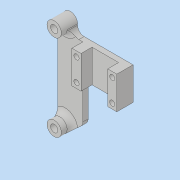
# Autodesk Inventor part: ribbonCableMount1
Saved by Autodesk Inventor 2017 (Build 210142000, 142)
## iProperties
Created: 2019-07-12
Part Number: ribbonCableMount1
Material: Generic
Document SubType Name: Modeling
Designer: techn
Density: 1 g/cm^3
Appearance: Default
Author: techn
Autodesk Inventor part; units mm, degrees
ref_plane "YZ Plane" through (0, 0, 0) normal (1, 0, 0) x (0, 1, 0)
ref_plane "XZ Plane" through (0, 0, 0) normal (0, 1, 0) x (-1, 0, 0)
ref_plane "XY Plane" through (0, 0, 0) normal (0, 0, 1) x (1, 0, 0)
sketch "Sketch1" plane through (0, 0, 0) normal (0, 0, 1) x (1, 0, 0)
  circle A0 centre (0, 0) radius 3.4925
  circle A1 centre (0, 41.91) radius 3.4925
  line L0 (0, 0) -> (-43.0857, 0) construction
  circle A2 centre (0, 41.91) radius 1.778
  circle A3 centre (0, 0) radius 1.778
  line L1 (3.4925, 41.91) -> (3.4925, 38.1)
  line L2 (3.4925, 38.1) -> (30.48, 38.1)
  line L3 (30.48, 38.1) -> (30.48, 22.225)
  line L4 (30.48, 22.225) -> (2.3101, -2.6193)
  line L5 (-3.4925, 41.91) -> (-3.4925, 0)
  dimension "d0" = 6.985
  dimension "d1" = 6.985
  dimension "d2" = 41.91
  dimension "d3" = 90
  dimension "d5" = 3.556
  dimension "d6" = 3.556
  dimension "d7" = 3.81
  dimension "d8" = 30.48
  dimension "d29" = 15.875
  constraints: 12 end point, 4 centre point, 4 point on circle, 4 tangent, 3 coincident, 2 perpendicular, 1 horizontal, 1 vertical
  measures "d0" diameter of A0
  measures "d1" diameter of A1
  measures "d2" distance of point (0, 0) A1.centre
  measures "d5" diameter of A2
  measures "d6" diameter of A3
  measures "d7" distance from line of L2 A1.centre
  measures "d8" distance from line of L3 A1.centre
  measures "d29" distance of L2.end L3.end
extrude "Extrusion1" add sketch "Sketch1" along normal blind 2.54
sketch "Sketch3" plane through (0, 0, 2.54) normal (0, 0, 1) x (1, 0, 0)
  circle A0 centre (0, 41.91) radius 1.778 construction
  circle A1 centre (0, 0) radius 1.778 construction
  arc A2 (-3.4925, 0) -> (2.3101, -2.6193) centre (0, 0) ccw construction
  line L0 (2.3101, -2.6193) -> (30.48, 22.225) construction
  line L1 (30.48, 22.225) -> (30.48, 38.1) construction
  line L2 (30.48, 38.1) -> (3.4925, 38.1) construction
  line L3 (3.4925, 38.1) -> (3.4925, 41.91) construction
  arc A3 (3.4925, 41.91) -> (-3.4925, 41.91) centre (0, 41.91) ccw construction
  line L4 (-3.4925, 41.91) -> (-3.4925, 0) construction
  line L5 (30.48, 22.225) -> (30.48, 38.1) projected
  line L6 (30.48, 38.1) -> (26.035, 38.1)
  line L7 (26.035, 38.1) -> (26.035, 22.225)
  line L8 (26.035, 22.225) -> (30.48, 22.225)
  line L9 (30.48, 22.225) -> (30.48, 38.1)
  line L10 (13.081, 38.1) -> (8.636, 38.1)
  line L11 (8.636, 38.1) -> (8.636, 22.225)
  line L12 (8.636, 22.225) -> (13.081, 22.225)
  line L13 (13.081, 22.225) -> (13.081, 38.1)
  line L14 (26.035, 22.225) -> (13.081, 22.225) construction
  dimension "d11" = 4.445
  dimension "d12" = 12.954
  constraints: 18 end point, 4 parallel, 2 collinear, 2 horizontal, 2 perpendicular, 2 point on line, 1 coincident
  measures "d11" distance of L7.end L8.end
  measures "d12" distance between parallel lines of L13 L7
extrude "Extrusion2" add sketch "Sketch3" along normal blind 5.334
fillet "Fillet1" radius 3.175 1 edges at (3.4925, 38.1, 1.27)
sketch "Sketch5" plane through (0, 0, 7.874) normal (0, 0, 1) x (1, 0, 0)
  circle A0 centre (10.8585, 35.56) radius 1.27
  circle A1 centre (10.8585, 24.765) radius 1.27
  circle A2 centre (28.2575, 35.56) radius 1.27
  circle A3 centre (28.2575, 24.765) radius 1.27
  line L0 (13.081, 38.1) -> (8.636, 38.1) construction
  line L1 (8.636, 38.1) -> (8.636, 22.225) construction
  line L2 (8.636, 22.225) -> (13.081, 22.225) construction
  line L3 (13.081, 22.225) -> (13.081, 38.1) construction
  line L4 (30.48, 38.1) -> (26.035, 38.1) construction
  line L5 (26.035, 38.1) -> (26.035, 22.225) construction
  line L6 (26.035, 22.225) -> (30.48, 22.225) construction
  line L7 (30.48, 22.225) -> (30.48, 38.1) construction
  point P0 (0, 0)
  point P1 (10.8585, 38.1)
  point P2 (28.2575, 38.1)
  dimension "d21" = 2.54
  dimension "d22" = 2.54
  dimension "d23" = 2.54
  dimension "d24" = 2.54
  dimension "d25" = 2.54
  dimension "d26" = 2.54
  constraints: 4 centre point, 4 vertical alignment, 2 horizontal alignment, 2 midpoint
  measures "d21" diameter of A0
  measures "d22" diameter of A1
  measures "d23" diameter of A2
  measures "d24" diameter of A3
  measures "d25" distance from line of L0 A0.centre
  measures "d26" distance from line of L2 A1.centre
extrude "Extrusion4" cut sketch "Sketch5" against normal through all
sketch "Sketch6" plane through (0, 0, 2.54) normal (0, 0, 1) x (1, 0, 0)
  circle A0 centre (0, 41.91) radius 1.778 projected
  arc A1 (3.4925, 41.91) -> (-3.4925, 41.91) centre (0, 41.91) ccw projected
  circle A2 centre (0, 0) radius 3.4925
  circle A3 centre (0, 41.91) radius 3.4925
  circle A4 centre (0, 0) radius 1.778 projected
  constraints: 2 coincident, 1 centre point, 1 horizontal alignment, 2 other
extrude "Extrusion5" add sketch "Sketch6" along normal up to surface (5.334 mm away)
fillet "Fillet3" radius 2.54 3 edges at (0, 38.4175, 2.54) (3.1832, -1.4369, 2.54) (0, 3.4925, 2.54)
sketch "Sketch7" plane through (0, 0, 2.54) normal (0, 0, 1) x (1, 0, 0)
  line L0 (5.9991, 0.6341) -> (30.48, 22.225) projected
  line L1 (30.48, 22.225) -> (8.636, 22.225)
  line L2 (8.636, 22.225) -> (8.636, 2.9598)
  point P0 (0, 0)
  constraints: 4 end point, 1 horizontal, 1 perpendicular, 1 point on line
extrude "Extrusion6" cut sketch "Sketch7" against normal blind 25.4
fillet "Fillet4" radius 3.175 2 edges at (8.636, 22.225, 1.27) (8.636, 2.9598, 1.27)
body "Solid1"
